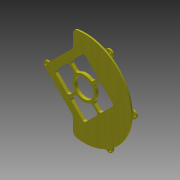
# Autodesk Inventor part: tapa
Saved by Autodesk Inventor 2015 (Build 190159000, 159)
## iProperties
Created: 2015-03-18
Part Number: tapa
Material: Genérico
Document SubType Name: Modeling
Designer: david_000
Density: 1 g/cm^3
Appearance: Valor por defecto
Author: david_000
Autodesk Inventor part; units mm, degrees
ref_plane "YZ Plane" through (0, 0, 0) normal (1, 0, 0) x (0, 1, 0)
ref_plane "XZ Plane" through (0, 0, 0) normal (0, 1, 0) x (-1, 0, 0)
ref_plane "XY Plane" through (0, 0, 0) normal (0, 0, 1) x (1, 0, 0)
sketch "Boceto1" plane through (0, 0, 0) normal (0, 1, 0) x (-1, 0, 0)
  circle A0 centre (0, 0) radius 120
  arc A1 (66.559, 99.8494) -> (0, -120) centre (0, 0) ccw
  line L0 (7.0711, -63.4624) -> (63.4624, -7.0711)
  line L1 (77.6045, 7.0711) -> (26.2589, 58.4167)
  line L2 (63.4624, 7.0711) -> (7.0711, 63.4624)
  spline S0 degree 3 poles (115, -17.0938) (114.7772, -17.0938) (114.5544, -17.0946) (109.1407, -17.1321) (103.9526, -17.5882) (93.3333, -19.3942) (87.9133, -20.8087) (79.4043, -23.8394) (76.2145, -25.1727) (69.1994, -28.5589) (65.4208, -30.709) (59.0238, -34.9471) (56.3389, -36.9347) (51.7862, -40.6903) (49.8726, -42.4032) (46.6161, -45.5673) (45.2434, -46.9877) (42.8987, -49.5764) (41.9074, -50.7272) (40.3572, -52.6253) (39.7791, -53.3569) (38.4933, -55.0437) (37.7932, -56.0049) (36.628, -57.6996) (36.1502, -58.4246) (35.2939, -59.8086) (34.9096, -60.4641) (34.3253, -61.5764) (34.1072, -62.0239) (33.7615, -62.8542) (33.6244, -63.2335) (33.4177, -64.0108) (33.3496, -64.4095) (33.3183, -65.2002) (33.3524, -65.59) (33.5018, -66.3538) (33.6151, -66.7279) (33.9933, -67.7556) (34.3036, -68.3919) (35.1043, -69.8899) (35.6207, -70.7385) (37.0242, -72.9169) (37.9488, -74.2226) (40.7678, -77.97) (42.7675, -80.3335) (46.9878, -84.8508) (49.2105, -87.0028) (56.1733, -93.117) (61.2161, -96.7416) (66.559, -99.8494) knots -14.899714 -14.899714 -14.899714 -14.899714 -14.832887 -14.832887 -13.275655 -13.275655 -11.601453 -11.601453 -10.565835 -10.565835 -9.264747 -9.264747 -8.26391 -8.26391 -7.494036 -7.494036 -6.901825 -6.901825 -6.446278 -6.446278 -6.16657 -6.16657 -5.809984 -5.809984 -5.549565 -5.549565 -5.321754 -5.321754 -5.172573 -5.172573 -5.051913 -5.051913 -4.931253 -4.931253 -4.814538 -4.814538 -4.697824 -4.697824 -4.486003 -4.486003 -4.18825 -4.18825 -3.708599 -3.708599 -2.781451 -2.781451 -1.854302 -1.854302 0 0 0 0
  spline S1 degree 3 poles (66.559, 99.8494) (65.4502, 99.2044) (64.3543, 98.5373) (60.5478, 96.1141) (57.9109, 94.2422) (53.4256, 90.7028) (51.5356, 89.088) (48.5657, 86.3408) (47.4456, 85.252) (45.025, 82.7779) (43.7379, 81.3794) (41.5415, 78.8356) (40.6134, 77.7063) (39.1126, 75.7783) (38.523, 74.9925) (37.3516, 73.3636) (36.7709, 72.5197) (35.77, 70.9731) (35.3407, 70.2765) (34.7151, 69.1682) (34.5001, 68.7671) (34.0885, 67.9287) (33.8931, 67.4907) (33.5675, 66.5901) (33.4379, 66.126) (33.2823, 64.9677) (33.3473, 64.2674) (33.6675, 63.0783) (33.8676, 62.5727) (34.3164, 61.5866) (34.5663, 61.1057) (35.1636, 60.0282) (35.5194, 59.4364) (37.067, 56.9795) (38.3646, 55.1819) (42.0672, 50.4272) (44.6123, 47.5785) (50.1315, 42.1) (53.1224, 39.4853) (65.3064, 30.1019) (75.6011, 24.7748) (95.7156, 18.551) (105.3578, 17.0938) (115, 17.0938) knots 6.581526 6.581526 6.581526 6.581526 6.966316 6.966316 7.935111 7.935111 8.680337 8.680337 9.148844 9.148844 9.718722 9.718722 10.15709 10.15709 10.451734 10.451734 10.75899 10.75899 11.004376 11.004376 11.140824 11.140824 11.284558 11.284558 11.428291 11.428291 11.635165 11.635165 11.797742 11.797742 11.960319 11.960319 12.167342 12.167342 12.831524 12.831524 13.975216 13.975216 15.164492 15.164492 18.5882 18.5882 21.480867 21.480867 21.480867 21.480867
  line L3 (149.8378, 65.1622) -> (98.9727, 14.2971)
  line L4 (77.6045, -7.0711) -> (26.2589, -58.4167)
  line L5 (23.3299, -65.4878) -> (23.3299, -89.0074)
  arc A2 (49.2901, -87.0086) -> (49.2901, 87.0085) centre (0, 0) ccw
  arc A3 (14.8111, 98.8971) -> (14.8111, -98.8971) centre (0, 0) ccw
  line L6 (23.3299, 89.0074) -> (23.3299, 65.4878)
  arc A4 (77.6045, -7.0711) -> (77.6045, 7.0711) centre (70.5335, 0) ccw
  arc A5 (23.3299, 65.4878) -> (26.2589, 58.4167) centre (33.3299, 65.4878) ccw
  arc A6 (23.3299, 89.0074) -> (14.8111, 98.8971) centre (13.3299, 89.0074) ccw
  arc A7 (14.8111, -98.8971) -> (23.3299, -89.0074) centre (13.3299, -89.0074) ccw
  arc A8 (26.2589, -58.4167) -> (23.3299, -65.4878) centre (33.3299, -65.4878) ccw
  point P0 (23.3299, -97.2405)
  point P1 (23.3299, 97.2405)
  dimension "d0" = 10
  dimension "d1" = 10
  constraints: 19 point on circle, 14 end point, 11 tangent, 9 centre point, 4 equal radius, 3 parallel, 2 coincident, 2 point on line, 6 other
  measures "d0" distance between parallel lines of L2 L1
  measures "d1" radius of A4
extrude "Extrusión1" add sketch "Boceto1" along normal blind 3 contours A4 L4 A8 L5 A7 A3 A6 L6 A5 L1
sketch "Boceto2" plane through (0, 3, 0) normal (0, 1, 0) x (1, 0, 0)
  circle A0 centre (0, 0) radius 100
  circle A1 centre (104, 0) radius 2
  circle A2 centre (104, 0) radius 4
  arc A3 (-14.8111, -98.8971) -> (-14.8111, 98.8971) centre (0, 0) ccw projected
  arc A4 (-14.8111, -98.8971) -> (-14.8111, 98.8971) centre (0, 0) ccw projected
  circle A5 centre (100, 0) radius 8
  circle A6 centre (52, 90.0666) radius 2
  circle A7 centre (50, 86.6025) radius 8
  circle A8 centre (-52, 90.0666) radius 2
  circle A9 centre (-50, 86.6025) radius 8
  circle A10 centre (-104, 0) radius 2
  circle A11 centre (-100, 0) radius 8
  circle A12 centre (-52, -90.0666) radius 2
  circle A13 centre (-50, -86.6025) radius 8
  circle A14 centre (52, -90.0666) radius 2
  circle A15 centre (50, -86.6025) radius 8
  dimension "d0" = 10
  dimension "d1" = 10
  dimension "d4" = 4
  dimension "d5" = 8
  dimension "d10" = 360
  constraints: 14 centre point, 2 coincident, 2 point on circle, 1 tangent, 25 other
  measures "d4" diameter of A1
  measures "d5" diameter of A2
extrude "Extrusión2" add sketch "Boceto2" along normal blind 3 contours A0 A5 | A2 A5 A0 | A0 A5 A2 | A2 | A7 A0 | A0 A7 | A15 A0 | A0 A15
fillet "Empalme1" radius 3 3 edges at (46, 3, 79.6743) (92, 3, 0) (46, 3, -79.6743)
fillet "Empalme2" radius 3 6 edges at (99.68, 4.5, 7.9936) (99.68, 4.5, -7.9936) (56.7627, 4.5, 82.3286) (42.9173, 4.5, 90.3222) (56.7627, 4.5, -82.3286) (42.9173, 4.5, -90.3222)
sketch "Boceto4" plane through (0, 3, 0) normal (0, 1, 0) x (1, 0, 0)
  arc A0 (-77.6045, 7.0711) -> (-77.6045, -7.0711) centre (-70.5335, 0) ccw projected
  circle A1 centre (-70.5335, 0) radius 10
  circle A2 centre (-84.5335, 0) radius 4
  circle A3 centre (-84.5335, 0) radius 2
  circle A4 centre (-80.5335, 0) radius 8
  point P0 (0, 0)
  dimension "d14" = 8
  dimension "d15" = 4
  constraints: 2 centre point, 2 coincident, 2 horizontal alignment, 5 other
  measures "d15" diameter of A3
extrude "Extrusión3" add sketch "Boceto4" along normal blind 3 contours A1 A4 A0 | A0 A2 A4 A1 | A2 | A0 A1 A4 A2
fillet "Empalme3" radius 3 2 edges at (-73.8423, 3, 4.385) (-73.8423, 3, -4.385)
fillet "Empalme4" radius 3 2 edges at (-77.3404, 4.5, -7.3352) (-77.3404, 4.5, 7.3352)
sketch "Boceto5" plane through (0, 0, 0) normal (0, -1, 0) x (1, 0, 0)
  circle A0 centre (0, 0) radius 135
  circle A1 centre (0, 0) radius 20
  line L0 (-26.4279, -29.9634) -> (-18.7718, -22.3074)
  line L1 (18.7718, -22.3074) -> (26.4279, -29.9634)
  line L2 (26.4279, -37.0345) -> (3.5355, -59.9269)
  line L3 (-26.4279, -37.0345) -> (-3.5355, -59.9269)
  arc A2 (-12.6969, -21.5357) -> (12.6969, -21.5357) centre (0, 0) ccw
  arc A3 (-3.5355, -59.9269) -> (3.5355, -59.9269) centre (0, -56.3913) ccw
  arc A4 (-26.4279, -29.9634) -> (-26.4279, -37.0345) centre (-22.8924, -33.499) ccw
  arc A5 (-12.6969, -21.5357) -> (-18.7718, -22.3074) centre (-15.2363, -25.8429) ccw
  arc A6 (18.7718, -22.3074) -> (12.6969, -21.5357) centre (15.2363, -25.8429) ccw
  arc A7 (26.4279, -37.0345) -> (26.4279, -29.9634) centre (22.8924, -33.499) ccw
  arc A8 (21.5357, -12.6969) -> (22.3074, -18.7718) centre (25.8429, -15.2363) ccw
  arc A9 (21.5357, -12.6969) -> (21.5357, 12.6969) centre (0, 0) ccw
  line L4 (29.9634, -26.4279) -> (22.3074, -18.7718)
  arc A10 (29.9634, -26.4279) -> (37.0345, -26.4279) centre (33.499, -22.8924) ccw
  arc A11 (37.0345, 26.4279) -> (29.9634, 26.4279) centre (33.499, 22.8924) ccw
  line L5 (37.0345, 26.4279) -> (59.9269, 3.5355)
  arc A12 (59.9269, -3.5355) -> (59.9269, 3.5355) centre (56.3913, 0) ccw
  line L6 (37.0345, -26.4279) -> (59.9269, -3.5355)
  line L7 (22.3074, 18.7718) -> (29.9634, 26.4279)
  arc A13 (22.3074, 18.7718) -> (21.5357, 12.6969) centre (25.8429, 15.2363) ccw
  arc A14 (12.6969, 21.5357) -> (18.7718, 22.3074) centre (15.2363, 25.8429) ccw
  arc A15 (12.6969, 21.5357) -> (-12.6969, 21.5357) centre (0, 0) ccw
  line L8 (26.4279, 29.9634) -> (18.7718, 22.3074)
  arc A16 (26.4279, 29.9634) -> (26.4279, 37.0345) centre (22.8924, 33.499) ccw
  arc A17 (-26.4279, 37.0345) -> (-26.4279, 29.9634) centre (-22.8924, 33.499) ccw
  line L9 (-26.4279, 37.0345) -> (-3.5355, 59.9269)
  arc A18 (3.5355, 59.9269) -> (-3.5355, 59.9269) centre (0, 56.3913) ccw
  line L10 (26.4279, 37.0345) -> (3.5355, 59.9269)
  line L11 (-18.7718, 22.3074) -> (-26.4279, 29.9634)
  arc A19 (-18.7718, 22.3074) -> (-12.6969, 21.5357) centre (-15.2363, 25.8429) ccw
  arc A20 (-21.5357, 12.6969) -> (-22.3074, 18.7718) centre (-25.8429, 15.2363) ccw
  arc A21 (-21.5357, 12.6969) -> (-21.5357, -12.6969) centre (0, 0) ccw
  line L12 (-29.9634, 26.4279) -> (-22.3074, 18.7718)
  arc A22 (-29.9634, 26.4279) -> (-37.0345, 26.4279) centre (-33.499, 22.8924) ccw
  arc A23 (-37.0345, -26.4279) -> (-29.9634, -26.4279) centre (-33.499, -22.8924) ccw
  line L13 (-37.0345, -26.4279) -> (-59.9269, -3.5355)
  arc A24 (-59.9269, 3.5355) -> (-59.9269, -3.5355) centre (-56.3913, 0) ccw
  line L14 (-37.0345, 26.4279) -> (-59.9269, 3.5355)
  line L15 (-22.3074, -18.7718) -> (-29.9634, -26.4279)
  arc A25 (-22.3074, -18.7718) -> (-21.5357, -12.6969) centre (-25.8429, -15.2363) ccw
  line L16 (63.4624, 7.0711) -> (7.0711, 63.4624)
  line L17 (-7.0711, 63.4624) -> (-63.4624, 7.0711)
  line L18 (-63.4624, -7.0711) -> (-7.0711, -63.4624)
  line L19 (63.4624, -7.0711) -> (7.0711, -63.4624)
  arc A26 (63.4624, -7.0711) -> (63.4624, 7.0711) centre (56.3913, 0) ccw
  arc A27 (7.0711, 63.4624) -> (-7.0711, 63.4624) centre (0, 56.3913) ccw
  arc A28 (-63.4624, 7.0711) -> (-63.4624, -7.0711) centre (-56.3913, 0) ccw
  arc A29 (-7.0711, -63.4624) -> (7.0711, -63.4624) centre (0, -56.3913) ccw
  line L20 (-65.1957, 8.8043) -> (-8.8043, 65.1957)
  arc A30 (8.8043, 65.1957) -> (-8.8043, 65.1957) centre (0, 56.3913) ccw
  line L21 (8.8043, 65.1957) -> (65.1957, 8.8043)
  arc A31 (65.1957, -8.8043) -> (65.1957, 8.8043) centre (56.3913, 0) ccw
  line L22 (65.1957, -8.8043) -> (8.8043, -65.1957)
  arc A32 (-8.8043, -65.1957) -> (8.8043, -65.1957) centre (0, -56.3913) ccw
  line L23 (-8.8043, -65.1957) -> (-65.1957, -8.8043)
  arc A33 (-65.1957, 8.8043) -> (-65.1957, -8.8043) centre (-56.3913, 0) ccw
  circle A34 centre (0, 0) radius 132
  point P0 (-29.9634, -33.499)
  point P1 (29.9634, -33.499)
  point P2 (-15.8213, -19.3568)
  point P3 (15.8213, -19.3568)
  point P4 (33.499, -29.9634)
  point P5 (33.499, 29.9634)
  point P6 (29.9634, 33.499)
  point P7 (-29.9634, 33.499)
  point P8 (-33.499, 29.9634)
  point P9 (-33.499, -29.9634)
  dimension "d22" = 20
  dimension "d23" = 20
  dimension "d24" = 5
  dimension "d25" = 360
  dimension "d26" = 5
  dimension "d27" = 5
  dimension "d28" = 5
  dimension "d29" = 10
  dimension "d30" = 2.4512
  dimension "d31" = 270
  dimension "d32" = 3
  constraints: 66 point on circle, 48 end point, 35 centre point, 18 point on line, 18 tangent, 7 equal radius, 5 coincident, 4 parallel, 2 perpendicular, 122 other
  measures "d22" distance of point (-29.963, -33.499) point (-15.821, -19.357)
  measures "d23" distance of point (15.821, -19.357) point (29.963, -33.499)
  measures "d24" radius of A3
  measures "d26" distance between parallel lines of L16 L10
  measures "d27" distance between parallel lines of L14 L17
  measures "d28" distance between parallel lines of L6 L19
  measures "d29" radius of A26
  measures "d30" distance between parallel lines of L17 L20
  measures "d31" diameter of A0
  measures "d32" radial gap between concentric circles of A0 A34
extrude "Extrusión4" cut sketch "Boceto5" against normal blind 3 contours A1 | L0 A5 A2 A6 L1 A7 L2 A3 L3 A4 | A9 A13 L7 A11 L5 A12 L6 A10 L4 A8 | A15 A19 L11 A17 L9 A18 L10 A16 L8 A14 | A21 A25 L15 A23 L13 A24 L14 A22 L12 A20
extrude "Extrusión5" add sketch "Boceto5" against normal blind 6 contours A26 L19 A29 L18 A28 L17 A27 L16
fillet "Empalme5" radius 3 16 edges at (66.3913, 3, 0) (35.2667, 3, 35.2667) (0, 3, 66.3913) (-35.2667, 3, 35.2667) (-66.3913, 3, 0) (-35.2667, 3, -35.2667) (0, 3, -66.3913) (35.2667, 3, -35.2667) (0, 6, -66.3913) (-35.2667, 6, -35.2667) (-66.3913, 6, 0) (-35.2667, 6, 35.2667) (0, 6, 66.3913) (35.2667, 6, 35.2667) (66.3913, 6, 0) (35.2667, 6, -35.2667)
